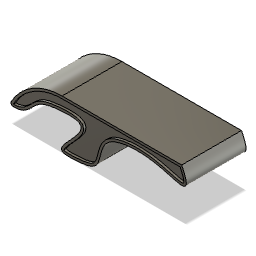
Bottle Opener v3 (Autodesk Fusion 360 design; units mm, degrees)
Autodesk Fusion 360 part; units mm, degrees
sketch "Sketch1" plane through (0, 0, 0) normal (0, 0, 1) x (1, 0, 0)
  line L0 (49.8303, 29.9197) -> (-0.1697, 29.9197)
  arc A0 (-0.1697, 29.9197) -> (-22.0765, 15.9797) centre (-0.1697, 5.7364) ccw
  spline S0 degree 5 poles (-22.0765, 15.9797) (-21.6945, 15.9199) (-20.9457, 15.83) (-19.8679, 15.7844) (-18.522, 15.9019) (-16.9894, 16.339) (-15.5998, 17.0431) (-14.3395, 17.9687) (-13.1852, 19.0361) (-12.1016, 20.1407) (-11.0369, 21.1798) (-9.9214, 22.0708) (-8.6595, 22.7796) (-7.1413, 23.3245) (-5.279, 23.7459) (-3.0413, 24.083) (-0.4829, 24.35) (2.2111, 24.5059) (4.7276, 24.4492) (6.7168, 24.0597) (7.8679, 23.2324) (7.9848, 21.9114) (7.077, 20.1315) (5.3966, 18.0334) (3.3366, 15.8168) (1.3565, 13.7048) (-0.104, 11.903) (-0.7034, 10.5631) (-0.2867, 9.7402) (1.0482, 9.363) (3.049, 9.2993) (5.3899, 9.4091) (7.7647, 9.6092) (9.9553, 9.913) (11.8179, 10.3855) (13.2816, 11.1113) (14.3426, 12.1587) (15.0606, 13.5435) (15.5529, 15.1975) (15.9684, 17.0015) (16.4622, 18.8146) (17.1715, 20.5024) (18.1872, 21.9708) (19.5408, 23.1817) (21.2221, 24.1333) (23.1917, 24.8472) (25.3941, 25.3541) (27.7723, 25.6778) (30.2774, 25.8256) (32.8646, 25.7982) (35.4909, 25.5957) (38.1122, 25.2258) (40.6807, 24.7112) (43.1425, 24.0961) (45.4339, 23.4558) (47.4826, 22.8959) (49.2144, 22.5352) (50.5592, 22.4933) (51.457, 22.8765) (51.8649, 23.7624) (51.7583, 25.1954) (51.2519, 26.7973) (50.6338, 28.2578) (50.1158, 29.3466) (49.8303, 29.9197) knots 0 0 0 0 0 0 0.01666667 0.03333333 0.05 0.06666667 0.08333333 0.1 0.11666667 0.13333333 0.15 0.16666667 0.18333333 0.2 0.21666667 0.23333333 0.25 0.26666667 0.28333333 0.3 0.31666667 0.33333333 0.35 0.36666667 0.38333333 0.4 0.41666667 0.43333333 0.45 0.46666667 0.48333333 0.5 0.51666667 0.53333333 0.55 0.56666667 0.58333333 0.6 0.61666667 0.63333333 0.65 0.66666667 0.68333333 0.7 0.71666667 0.73333333 0.75 0.76666667 0.78333333 0.8 0.81666667 0.83333333 0.85 0.86666667 0.88333333 0.9 0.91666667 0.93333333 0.95 0.96666667 0.98333333 1 1 1 1 1 1
  spline S1 degree 3 poles (-20.5245, 16.8338) (-18.9017, 16.7844) (-17.5543, 17.1434) (-16.3465, 17.8372) (-14.9711, 18.6271) (-13.7773, 19.9002) (-12.5104, 21.1281) (-11.4446, 22.161) (-10.2842, 23.1178) (-8.7583, 23.7584) (-7.4276, 24.3171) (-5.8232, 24.6734) (-3.8599, 24.9535) (-2.0973, 25.2051) (-0.0266, 25.4078) (1.984, 25.4495) (3.5434, 25.4818) (5.0311, 25.4181) (6.2539, 25.0857) (7.0374, 24.8727) (7.7502, 24.545) (8.2505, 23.9357) (8.6471, 23.4528) (8.8383, 22.7946) (8.7988, 22.1704) (8.7305, 21.0919) (8.1515, 20.0782) (7.3661, 18.9901) (6.1105, 17.2502) (4.2179, 15.3338) (2.7502, 13.7018) (1.9763, 12.8412) (1.328, 12.0608) (0.9492, 11.4744) (0.6926, 11.077) (0.5723, 10.769) (0.5504, 10.6477) knots 0.013727 0.013727 0.013727 0.013727 0.063969 0.063969 0.063969 0.121179 0.121179 0.121179 0.169303 0.169303 0.169303 0.211274 0.211274 0.211274 0.248957 0.248957 0.248957 0.278182 0.278182 0.278182 0.296905 0.296905 0.296905 0.311745 0.311745 0.311745 0.337389 0.337389 0.337389 0.378389 0.378389 0.378389 0.400008 0.400008 0.400008 0.414658 0.414658 0.414658 0.414658
  spline S2 degree 3 poles (0.5504, 10.6477) (0.6314, 10.6011) (0.8203, 10.5285) (1.0961, 10.4744) (1.9273, 10.3116) (3.4548, 10.3187) (5.0208, 10.4109) (6.7859, 10.515) (8.6078, 10.6982) (10.0271, 11.0081) (11.3064, 11.2873) (12.2369, 11.6776) (12.871, 12.2134) (13.4995, 12.7445) (13.9149, 13.4673) (14.262, 14.4801) (14.7777, 15.9846) (15.0844, 18.0339) (15.8795, 19.9128) (16.4954, 21.3681) (17.4441, 22.7026) (18.7404, 23.707) (20.9217, 25.3973) (23.9547, 26.2195) (27.2939, 26.5863) (30.4461, 26.9326) (33.9039, 26.8301) (37.2728, 26.3333) (40.1778, 25.9049) (43.0267, 25.1545) (45.4093, 24.5028) (46.8859, 24.0989) (48.1849, 23.7527) (49.1334, 23.6214) (49.81, 23.5277) (50.295, 23.5658) (50.4918, 23.6359) (50.6368, 23.6875) (50.6367, 23.6968) (50.6781, 23.7784) (50.7313, 23.883) (50.8054, 24.2265) (50.704, 24.8405) (50.5557, 25.7387) (50.0654, 27.131) (49.2063, 28.9197) knots 0.435332 0.435332 0.435332 0.435332 0.446723 0.446723 0.446723 0.48105 0.48105 0.48105 0.519739 0.519739 0.519739 0.55461 0.55461 0.55461 0.58918 0.58918 0.58918 0.640532 0.640532 0.640532 0.680309 0.680309 0.680309 0.747246 0.747246 0.747246 0.810435 0.810435 0.810435 0.864922 0.864922 0.864922 0.898692 0.898692 0.898692 0.922783 0.922783 0.922783 0.940535 0.940535 0.940535 0.963315 0.963315 0.963315 0.996634 0.996634 0.996634 0.996634
  line L1 (49.2063, 28.9197) -> (-0.1697, 28.9197)
  arc A1 (-0.1697, 28.9197) -> (-20.5245, 16.8338) centre (-0.1697, 5.7364) ccw
  point P0 (-15.0734, 17.4652)
  point P1 (-10.3439, 21.699)
  point P2 (-1.3247, 24.2456)
  point P3 (7.8006, 22.2295)
  point P4 (-0.4336, 10.8262)
  point P5 (14.1789, 12.1391)
  point P6 (16.9712, 19.9057)
  point P7 (50.9865, 22.7601)
  point P8 (24.884, 25.2005)
  point P9 (42.0735, 24.3517)
  point P10 (4.8749, 9.401)
  dimension "d2" = 50
  dimension "d10" = -1
  constraint horizontal L0
  constraint tangent L0 A0
  measures "d2" distance of L0.start L0.end
extrude "Extrude1" add sketch "Sketch1" along normal blind 25 contours L0 A0 S0 | S1 S2 L1 A1
ref_plane "WorkPlane1" through (14.8469, 19.6301, 12.5) normal (0, 0, 1) x (1, 0, 0)
sketch "Sketch2" plane through (14.8393, 19.5212, 12.5) normal (0, 0, 1) x (1, 0, 0)
  line L0 (-18.7924, -5.8475) -> (-0.7924, -5.8475)
  line L1 (-0.7924, -5.8475) -> (-0.7924, -7.2475)
  line L2 (-0.7924, -7.2475) -> (-18.7924, -7.2475)
  line L3 (-18.7924, -7.2475) -> (-18.7924, -5.8475)
  dimension "d5" = 18
  dimension "d6" = 1.4
  constraint horizontal L0
  constraint vertical L1
  constraint horizontal L2
  constraint vertical L3
  measures "d5" distance of L0.start L0.end
  measures "d6" distance of L0.start L2.end
extrude "Extrude2" cut sketch "Sketch2" along normal mid plane 18
sketch "Sketch3" plane through (0, 0, 0) normal (0, 0, 1) x (1, 0, 0)
sketch "Sketch4" plane through (0, 0, 0) normal (0, 0, 1) x (1, 0, 0)
sketch "Sketch5" plane through (0, 0, 0) normal (0, 0, 1) x (1, 0, 0)
extrude "Extrude3" cut sketch "Sketch1" along normal blind 1 contours S1 S2 L1 A1
sketch "Sketch6" plane through (0, 0, 25) normal (0, 0, 1) x (1, 0, 0)
  spline S0 degree 5 poles (-22.0765, 15.9797) (-21.6945, 15.9199) (-20.9457, 15.83) (-19.8679, 15.7844) (-18.522, 15.9019) (-16.9894, 16.339) (-15.5998, 17.0431) (-14.3395, 17.9687) (-13.1852, 19.0361) (-12.1016, 20.1407) (-11.0369, 21.1798) (-9.9214, 22.0708) (-8.6595, 22.7796) (-7.1413, 23.3245) (-5.279, 23.7459) (-3.0413, 24.083) (-0.4829, 24.35) (2.2111, 24.5059) (4.7276, 24.4492) (6.7168, 24.0597) (7.8679, 23.2324) (7.9848, 21.9114) (7.077, 20.1315) (5.3966, 18.0334) (3.3366, 15.8168) (1.3565, 13.7048) (-0.104, 11.903) (-0.7034, 10.5631) (-0.2867, 9.7402) (1.0482, 9.363) (3.049, 9.2993) (5.3899, 9.4091) (7.7647, 9.6092) (9.9553, 9.913) (11.8179, 10.3855) (13.2816, 11.1113) (14.3426, 12.1587) (15.0606, 13.5435) (15.5529, 15.1975) (15.9684, 17.0015) (16.4622, 18.8146) (17.1715, 20.5024) (18.1872, 21.9708) (19.5408, 23.1817) (21.2221, 24.1333) (23.1917, 24.8472) (25.3941, 25.3541) (27.7723, 25.6778) (30.2774, 25.8256) (32.8646, 25.7982) (35.4909, 25.5957) (38.1122, 25.2258) (40.6807, 24.7112) (43.1425, 24.0961) (45.4339, 23.4558) (47.4826, 22.8959) (49.2144, 22.5352) (50.5592, 22.4933) (51.457, 22.8765) (51.8649, 23.7624) (51.7583, 25.1954) (51.2519, 26.7973) (50.6338, 28.2578) (50.1158, 29.3466) (49.8303, 29.9197) knots 0 0 0 0 0 0 0.01666667 0.03333333 0.05 0.06666667 0.08333333 0.1 0.11666667 0.13333333 0.15 0.16666667 0.18333333 0.2 0.21666667 0.23333333 0.25 0.26666667 0.28333333 0.3 0.31666667 0.33333333 0.35 0.36666667 0.38333333 0.4 0.41666667 0.43333333 0.45 0.46666667 0.48333333 0.5 0.51666667 0.53333333 0.55 0.56666667 0.58333333 0.6 0.61666667 0.63333333 0.65 0.66666667 0.68333333 0.7 0.71666667 0.73333333 0.75 0.76666667 0.78333333 0.8 0.81666667 0.83333333 0.85 0.86666667 0.88333333 0.9 0.91666667 0.93333333 0.95 0.96666667 0.98333333 1 1 1 1 1 1
  line L0 (49.8303, 29.9197) -> (-0.1697, 29.9197)
  arc A0 (-0.1697, 29.9197) -> (-22.0765, 15.9797) centre (-0.1697, 5.7364) ccw
  spline S1 degree 3 poles (-20.5245, 16.8338) (-18.9017, 16.7844) (-17.5543, 17.1434) (-16.3465, 17.8372) (-14.9711, 18.6271) (-13.7773, 19.9002) (-12.5104, 21.1281) (-11.4446, 22.161) (-10.2842, 23.1178) (-8.7583, 23.7584) (-7.4276, 24.3171) (-5.8232, 24.6734) (-3.8599, 24.9535) (-2.0973, 25.2051) (-0.0266, 25.4078) (1.984, 25.4495) (3.5434, 25.4818) (5.0311, 25.4181) (6.2539, 25.0857) (7.0374, 24.8727) (7.7502, 24.545) (8.2505, 23.9357) (8.6471, 23.4528) (8.8383, 22.7946) (8.7988, 22.1704) (8.7305, 21.0919) (8.1515, 20.0782) (7.3661, 18.9901) (6.1105, 17.2502) (4.2179, 15.3338) (2.7502, 13.7018) (1.9763, 12.8412) (1.328, 12.0608) (0.9492, 11.4744) (0.6926, 11.077) (0.5723, 10.769) (0.5504, 10.6477) knots 0.013727 0.013727 0.013727 0.013727 0.063969 0.063969 0.063969 0.121179 0.121179 0.121179 0.169303 0.169303 0.169303 0.211274 0.211274 0.211274 0.248957 0.248957 0.248957 0.278182 0.278182 0.278182 0.296905 0.296905 0.296905 0.311745 0.311745 0.311745 0.337389 0.337389 0.337389 0.378389 0.378389 0.378389 0.400008 0.400008 0.400008 0.414658 0.414658 0.414658 0.414658
  spline S2 degree 3 poles (0.5504, 10.6477) (0.6314, 10.6011) (0.8203, 10.5285) (1.0961, 10.4744) (1.9273, 10.3116) (3.4548, 10.3187) (5.0208, 10.4109) (6.7859, 10.515) (8.6078, 10.6982) (10.0271, 11.0081) (11.3064, 11.2873) (12.2369, 11.6776) (12.871, 12.2134) (13.4995, 12.7445) (13.9149, 13.4673) (14.262, 14.4801) (14.7777, 15.9846) (15.0844, 18.0339) (15.8795, 19.9128) (16.4954, 21.3681) (17.4441, 22.7026) (18.7404, 23.707) (20.9217, 25.3973) (23.9547, 26.2195) (27.2939, 26.5863) (30.4461, 26.9326) (33.9039, 26.8301) (37.2728, 26.3333) (40.1778, 25.9049) (43.0267, 25.1545) (45.4093, 24.5028) (46.8859, 24.0989) (48.1849, 23.7527) (49.1334, 23.6214) (49.81, 23.5277) (50.295, 23.5658) (50.4918, 23.6359) (50.6368, 23.6875) (50.6367, 23.6968) (50.6781, 23.7784) (50.7313, 23.883) (50.8054, 24.2265) (50.704, 24.8405) (50.5557, 25.7387) (50.0654, 27.131) (49.2063, 28.9197) knots 0.435332 0.435332 0.435332 0.435332 0.446723 0.446723 0.446723 0.48105 0.48105 0.48105 0.519739 0.519739 0.519739 0.55461 0.55461 0.55461 0.58918 0.58918 0.58918 0.640532 0.640532 0.640532 0.680309 0.680309 0.680309 0.747246 0.747246 0.747246 0.810435 0.810435 0.810435 0.864922 0.864922 0.864922 0.898692 0.898692 0.898692 0.922783 0.922783 0.922783 0.940535 0.940535 0.940535 0.963315 0.963315 0.963315 0.996634 0.996634 0.996634 0.996634
  line L1 (49.2063, 28.9197) -> (-0.1697, 28.9197)
  arc A1 (-0.1697, 28.9197) -> (-20.5245, 16.8338) centre (-0.1697, 5.7364) ccw
  dimension "d13" = -1
extrude "Extrude4" cut sketch "Sketch6" against normal blind 1 contours S1 S2 L1 A1
fillet "Fillet1" radius 1 1 edges at (-22.0765, 15.9797, 12.5)
